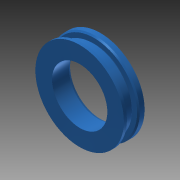
# Autodesk Inventor part: pully 16mmx30mmx6mm
Saved by Autodesk Inventor 2013 (Build 170138000, 138)
## iProperties
Created: 2016-11-25
Part Number: pully 16mmx30mmx6mm
Material: Generic
Document SubType Name: Modeling
Designer: hdv
Density: 1 g/cm^3
Author: hdv
Autodesk Inventor part; units mm, degrees
ref_plane "YZ Plane" through (0, 0, 0) normal (1, 0, 0) x (0, 1, 0)
ref_plane "XZ Plane" through (0, 0, 0) normal (0, 1, 0) x (-1, 0, 0)
ref_plane "XY Plane" through (0, 0, 0) normal (0, 0, 1) x (1, 0, 0)
sketch "Sketch1" plane through (0, 0, 0) normal (0, 0, 1) x (1, 0, 0)
  line L0 (11.1, 0) -> (17.1, 0)
  line L1 (17.1, 0) -> (17.1, 8) construction
  line L2 (17.1, 8) -> (11.1, 8) construction
  line L3 (11.1, 8) -> (11.1, 0) construction
  line L4 (0, 0) -> (0, 7.3935) construction
  line L5 (17.1, 8) -> (17.1, 6.8284)
  line L6 (17.1, 1.1716) -> (17.1, 0)
  circle A0 centre (18.1, 4) radius 3
  line L7 (15.1, 5.6) -> (15.1, 2.4) construction
  line L8 (15.1, 2.4) -> (16.4287, 1.5087)
  line L9 (14.7, 5.6) -> (16.6, 5.6)
  line L10 (16.6, 5.6) -> (17.1, 6.1)
  line L11 (17.1, 6.1) -> (17.1, 6.8284)
  line L12 (14.7, 5.6) -> (15.1, 5.1)
  line L13 (15.1, 5.1) -> (15.1, 2.4)
  line L14 (11.7, 8) -> (11.1, 7)
  line L15 (11.1, 0.4) -> (10.7, 0)
  line L16 (10.7, 0) -> (11.1, 0)
  line L17 (11.7, 8) -> (17.1, 8)
  line L18 (11.1, 7) -> (11.1, 0.4)
  point P0 (17.1, 4)
  point P1 (15.5286, 5.5452)
  point P2 (15.5286, 2.4548)
  point P3 (15.1, 4)
  point P4 (16.3509, 6.4373)
  dimension "d13" = 6
  dimension "d6" = 8
  dimension "d7" = 11.1
  dimension "d12" = 1
  dimension "d14" = 6
  dimension "d17" = 3.2
  dimension "d18" = 1.9
  dimension "d19" = 135
  dimension "d24" = 0.5
  dimension "d25" = 0.5
  dimension "d27" = 0.6
  dimension "d28" = 1
  dimension "d29" = 0.4
  dimension "d30" = 0.4
  constraints: 38 end point, 8 point on line, 4 collinear, 4 perpendicular, 3 vertical, 2 horizontal alignment, 2 midpoint, 2 parallel, 1 coincident, 1 horizontal, 10 other
  measures "d6" distance of L1.end L0.end
  measures "d7" distance from line of L3 point (0, 0)
  measures "d12" distance of point (18.1, 4) point (17.1, 4)
  measures "d14" distance of L0.start L0.end
  measures "d17" distance of L7.start L7.end
  measures "d18" distance of L9.start L9.end
  measures "d19" angle of L10 L9
  measures "d24" horizontal distance of L1.end L9.end
  measures "d25" distance from line of L9 L12.end
  measures "d27" distance of L2.end L14.start
  measures "d28" distance of L14.end L2.end
  measures "d29" distance of L15.start L0.start
  measures "d30" distance of L15.end L0.start
revolve "Revolution1" add sketch "Sketch1" angle 360 about axis through (0, 0, 0) along (0, 1, 0) picked at (16.0469, 5.7737) contours L16 L15 L18 L14 L17 L5 A0 L9 L12 L13 L8 L6 L0 | L11 L10 L9 A0
body "Solid1"
